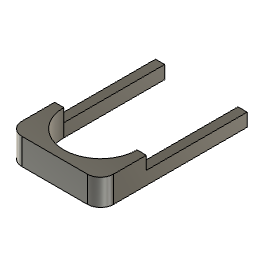
tube_case_front (Autodesk Fusion 360 design; units mm, degrees)
Autodesk Fusion 360 part; units mm, degrees
sketch "Sketch1" plane through (0, 0, 0) normal (0, 0, 1) x (1, 0, 0)
  circle A0 centre (0, 0) radius 14
  line L0 (14, 0) -> (-14, 0)
  line L1 (-17.5, 0) -> (-17.5, -17.5)
  line L2 (-17.5, -17.5) -> (17.5, -17.5)
  line L3 (17.5, -17.5) -> (17.5, 0)
  line L4 (-17.5, 0) -> (-17.5, 38.5)
  line L5 (17.5, 0) -> (17.5, 38.5)
  line L6 (-17.5, 0) -> (-17.5, 38.5)
  line L7 (-17.5, 38.5) -> (-14, 38.5)
  line L8 (-14, 38.5) -> (-14, 0)
  line L9 (17.5, 0) -> (17.5, 38.5)
  line L10 (17.5, 38.5) -> (14, 38.5)
  line L11 (14, 38.5) -> (14, 0)
  line L12 (-14, 38.5) -> (14, 38.5)
  arc A1 (-17.5, 0.003) -> (-17.5, -0.003) centre (0, 0) ccw
  line L13 (-17.5, 0) -> (-14, 0)
  line L14 (17.5, 0) -> (14, 0)
  dimension "d1" = 28
  dimension "d2" = 35
  dimension "d3" = 35
  dimension "d4" = 17.5
  dimension "d5" = 38.5
  dimension "d6" = 38.5
  constraint coincident A0.centre A1.centre
  constraint horizontal L0
  constraint vertical L1
  constraint horizontal L2
  constraint vertical L3
  constraint coincident L3.end A1
  constraint perpendicular L0 L4
  constraint perpendicular L0 L5
  constraint vertical L6
  constraint horizontal L7
  constraint vertical L8
  constraint coincident A0 L0.end
  constraint vertical L9
  constraint horizontal L10
  constraint vertical L11
  constraint coincident A0 L0.start
  constraint coincident L4 A1.start
  constraint coincident L1 A1.end
  constraint perpendicular L8 L13
  constraint perpendicular L11 L14
  measures "d1" diameter of A0
  measures "d2" diameter of A1
  measures "d3" distance of L3.end L1.start
  measures "d4" distance of L3.end L2.end
  measures "d5" distance of L1.start L4.end
  measures "d6" distance of L3.end L5.end
extrude "Extrude1" add sketch "Sketch1" along normal blind 10 contours A0 L1 L2 L3 A1 L13 L14
extrude "Extrude2" add sketch "Sketch1" along normal blind 5 contours L5 L9 L10 L11 L14 | L4 L6 L7 L8 A1 L13
fillet "Fillet1" radius 5 2 edges at (-17.5, -17.5, 5) (17.5, -17.5, 5)
